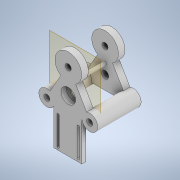
# Autodesk Inventor part: Platform 1 piece
Saved by Autodesk Inventor 2021 (Build 250183000, 183)
## iProperties
Created: 2021-04-26
Part Number: Platform 1 piece
Material: Generic
Document SubType Name: Modeling
Designer: Olivi
Density: 1 g/cm^3
Appearance: Default
Author: Olivi
Autodesk Inventor part; units mm, degrees
ref_plane "YZ Plane" through (0, 0, 0) normal (1, 0, 0) x (0, 1, 0)
ref_plane "XZ Plane" through (0, 0, 0) normal (0, 1, 0) x (-1, 0, 0)
ref_plane "XY Plane" through (0, 0, 0) normal (0, 0, 1) x (1, 0, 0)
sketch "Sketch1" plane through (0, 0, 0) normal (0, 0, 1) x (1, 0, 0)
  line L0 (0, 0) -> (70, 0)
  line L1 (70, 0) -> (35, 60.6218)
  line L2 (35, 60.6218) -> (0, 0)
  circle A0 centre (35, 20.5961) radius 5.5
  circle A1 centre (35, 57.6961) radius 20
  point P0 (46.2401, 41.1534)
  point P1 (23.7599, 41.1534)
  dimension "d0" = 70
  dimension "d1" = 70
  dimension "d2" = 60
  dimension "d3" = 11
  dimension "d4" = 37.1
  dimension "d5" = 40
  constraints: 6 end point, 2 centre point, 1 horizontal
  measures "d0" distance of L0.start L0.end
  measures "d1" distance of L0.end L1.end
  measures "d2" angle of L1 L0
  measures "d3" diameter of A0
  measures "d4" distance of A0.centre A1.centre
  measures "d5" diameter of A1
extrude "Extrusion1" add sketch "Sketch1" along normal blind 65.1
ref_plane "Work Plane1" through (0, 0, 55.1) normal (0, 0, 1) x (1, 0, 0)
sketch "Sketch2" plane through (0, 0, 55.1) normal (0, 0, 1) x (1, 0, 0)
  line L0 (14.3119, 82.6705) -> (-13.7787, 82.6705)
  line L1 (-13.7787, 82.6705) -> (-13.7787, -9.2093)
  line L2 (-13.7787, -9.2093) -> (82.9291, -9.2093)
  line L3 (82.9291, -9.2093) -> (82.9291, 82.6705)
  line L4 (82.9291, 82.6705) -> (14.3119, 82.6705)
  point P0 (0, 0)
  constraints: 10 end point, 4 perpendicular, 1 horizontal, 1 point on line
extrude "Extrusion2" cut sketch "Sketch2" against normal blind 45.2
sketch "Sketch3" plane through (0, 0, 65.1) normal (0, 0, 1) x (1, 0, 0)
  arc A0 (46.2401, 41.1534) -> (23.7599, 41.1534) centre (35, 57.6961) ccw projected
  circle A1 centre (35, 57.6961) radius 4.5
  point P0 (0, 0)
  dimension "d11" = 9
  constraints: 1 centre point, 1 coincident
  measures "d11" diameter of A1
extrude "Extrusion3" cut sketch "Sketch3" against normal through all
pattern_circular "Circular Pattern1" count 3 over 360 about axis through (35, 20.5961, 0) along (0, 0, 1) of "Extrusion3"
sketch "Sketch4" plane through (0, 0, 65.1) normal (0, 0, 1) x (1, 0, 0)
  arc A0 (6.8784, 0) -> (3.7314, 6.463) centre (2.8705, 2.0461) ccw projected
  circle A1 centre (2.8705, 2.0461) radius 4.5
  circle A2 centre (2.8705, 2.0461) radius 12
  arc A3 (66.2686, 6.463) -> (63.1216, 0) centre (67.1295, 2.0461) ccw projected
  circle A4 centre (67.1295, 2.0461) radius 4.5
  circle A5 centre (67.1295, 2.0461) radius 12
  point P0 (0, 0)
  point P1 (63.1216, 0)
  point P2 (66.2686, 6.463)
  point P3 (6.8784, 0)
  point P4 (3.7314, 6.463)
  dimension "d17" = 24
  dimension "d18" = 24
  constraints: 4 centre point, 4 coincident
  measures "d17" diameter of A2
  measures "d18" diameter of A5
extrude "Extrusion4" add sketch "Sketch4" against normal blind 65.1
sketch "Sketch5" plane through (0, 0, 65.1) normal (0, 0, 1) x (1, 0, 0)
  line L0 (23.7599, 41.1534) -> (7.5589, 13.0923) projected
  line L1 (13.3053, -58) -> (55.3053, -58)
  line L2 (55.3053, -58) -> (55.3053, 0)
  line L3 (14.6947, 0) -> (55.3053, 0) projected
  line L4 (13.3053, -58) -> (13.3053, 0)
  line L5 (13.3053, 0) -> (15.6594, 0)
  point P0 (0, 0)
  dimension "d22" = 42
  dimension "d24" = 0
  dimension "d26" = 58
  constraints: 8 end point, 2 point on line, 1 perpendicular, 1 vertical
  measures "d22" distance of L1.start L1.end
  measures "d24" distance from line of L3.end L2
  measures "d26" distance of L1.end L2.end
extrude "Extrusion5" add sketch "Sketch5" against normal blind 6
sketch "Sketch6" plane through (0, 0, 65.1) normal (0, 0, 1) x (1, 0, 0)
  circle A0 centre (35, 20.5961) radius 5.5 projected
  circle A1 centre (35, 20.5961) radius 11
  point P0 (0, 0)
  dimension "d29" = 22
  constraints: 1 centre point, 1 coincident
  measures "d29" diameter of A1
extrude "Extrusion6" cut sketch "Sketch6" against normal blind 8
sketch "Sketch7" plane through (35, 20.5961, 57.1) normal (0, 0, 1) x (1, 0, 0)
  circle A0 centre (-0.0422, -7.6) radius 1.25
  circle A1 centre (0, 0) radius 5.5 projected
  point P0 (-35, -20.5961)
  dimension "d32" = 2.5
  dimension "d33" = 7.6
  constraints: 1 centre point
  measures "d32" diameter of A0
  measures "d33" vertical distance of A0.centre A1.centre
extrude "Extrusion7" cut sketch "Sketch7" against normal blind 5 contours A0
sketch "Sketch8" plane through (0, 0, 65.1) normal (0, 0, 1) x (1, 0, 0)
  line L0 (18.1078, -53.5536) -> (18.1078, -11.6696)
  line L1 (18.1078, -11.6696) -> (21.3078, -11.6696)
  line L2 (21.3078, -11.6696) -> (21.3078, -53.5536)
  line L3 (21.3078, -53.5536) -> (18.1078, -53.5536)
  line L4 (51.8078, -11.6696) -> (51.8078, -53.5536)
  line L5 (51.8078, -53.5536) -> (48.6078, -53.5536)
  line L6 (48.6078, -53.5536) -> (48.6078, -11.6696)
  line L7 (48.6078, -11.6696) -> (51.8078, -11.6696)
  circle A0 centre (34.9578, 12.9961) radius 1.25 projected
  arc A1 (48.6078, -53.5536) -> (51.8078, -53.5536) centre (50.2078, -53.5536) ccw
  arc A2 (51.8078, -11.6696) -> (48.6078, -11.6696) centre (50.2078, -11.6696) ccw
  arc A3 (18.1078, -53.5536) -> (21.3078, -53.5536) centre (19.7078, -53.5536) ccw
  arc A4 (21.3078, -11.6696) -> (18.1078, -11.6696) centre (19.7078, -11.6696) ccw
  point P0 (0, 0)
  point P1 (21.7083, -32.6116)
  point P2 (52.2083, -32.6116)
  dimension "d36" = 3.2
  dimension "d37" = 3.2
  dimension "d38" = 30.5
  dimension "d41" = 13.65
  dimension "d42" = 13.65
  constraints: 16 end point, 8 point on circle, 8 tangent, 6 perpendicular, 4 centre point, 4 point on line, 1 vertical
  measures "d36" distance of L0.end L1.end
  measures "d37" distance of L4.end L5.end
  measures "d38" distance of point (21.708, -32.612) point (52.208, -32.612)
  measures "d41" distance from line of L2 A0.centre
  measures "d42" distance from line of L6 A0.centre
extrude "Extrusion8" cut sketch "Sketch8" against normal blind 10 contours L0 L1 L2 L3 | L3 A3 | A4 L1 | L4 L5 L6 L7 | L7 A2 | A1 L5
sketch "Sketch9" plane through (0, 0, 65.1) normal (0, 0, 1) x (1, 0, 0)
  circle A0 centre (35, 28.1961) radius 1.1
  circle A1 centre (35, 20.5961) radius 5.5 projected
  point P0 (0, 0)
  dimension "d45" = 2.2
  dimension "d46" = 7.6
  constraints: 1 centre point
  measures "d45" diameter of A0
  measures "d46" distance of A1.centre A0.centre
extrude "Extrusion9" cut sketch "Sketch9" against normal blind 10 contours A0
sketch "Sketch10" plane through (0, 0, 65.1) normal (0, 0, 1) x (1, 0, 0)
  circle A0 centre (35, 35.2401) radius 2.5
  point P0 (0, 0)
  dimension "d49" = 5
  constraints: 1 centre point
  measures "d49" diameter of A0
extrude "Extrusion10" add sketch "Sketch10" against normal blind 65
body "Solid1"
